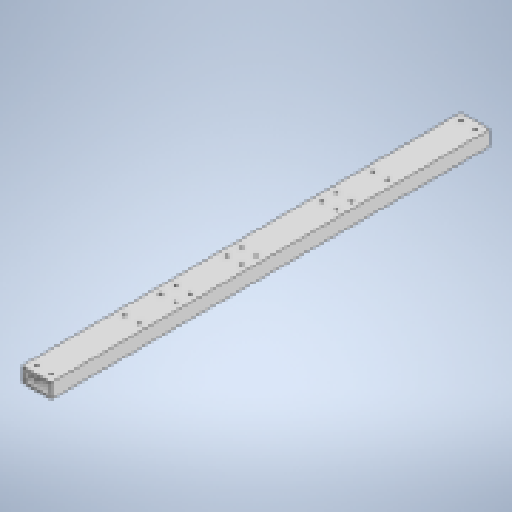
# Autodesk Inventor part: HorizontalSupportBar
Saved by Autodesk Inventor 2023 (Build 270158000, 158)
## iProperties
Created: 2022-07-13
Part Number: HorizontalSupportBar
Material: Generic
Document SubType Name: Modeling
Designer: Pratyush
Density: 1 g/cm^3
Appearance: Default
Author: Pratyush
Autodesk Inventor part; units mm, degrees
ref_plane "YZ Plane" through (0, 0, 0) normal (1, 0, 0) x (0, 1, 0)
ref_plane "XZ Plane" through (0, 0, 0) normal (0, 1, 0) x (-1, 0, 0)
ref_plane "XY Plane" through (0, 0, 0) normal (0, 0, 1) x (1, 0, 0)
sketch "Sketch1" plane through (0, 0, 0) normal (0, 0, 1) x (1, 0, 0)
  line L0 (-22.0343, 7.401) -> (28.7657, 7.401)
  line L1 (28.7657, 7.401) -> (28.7657, -17.999)
  line L2 (28.7657, -17.999) -> (-22.0343, -17.999)
  line L3 (-22.0343, -17.999) -> (-22.0343, 7.401)
  line L4 (-18.8593, 4.226) -> (25.5907, 4.226)
  line L5 (25.5907, 4.226) -> (25.5907, -14.824)
  line L6 (25.5907, -14.824) -> (-18.8593, -14.824)
  line L7 (-18.8593, -14.824) -> (-18.8593, 4.226)
  point P0 (0, 0)
  dimension "d0" = 50.8
  dimension "d1" = 25.4
  dimension "d2" = 3.175
  dimension "d3" = 3.175
  dimension "d4" = 3.175
  dimension "d5" = 3.175
  constraints: 16 end point, 4 parallel, 2 horizontal, 2 perpendicular
  measures "d0" distance of L0.start L0.end
  measures "d1" distance of L2.end L0.start
  measures "d2" distance between parallel lines of L0 L4
  measures "d3" distance between parallel lines of L2 L6
  measures "d4" distance between parallel lines of L1 L5
  measures "d5" distance between parallel lines of L3 L7
extrude "Extrusion1" add sketch "Sketch1" along normal mid plane 762
sketch "Sketch2" plane through (-22.0343, 7.401, 381) normal (0, 1, 0) x (1, 0, 0)
  line L0 (50.8, 0) -> (0, 0) projected
  line L1 (0, 762) -> (0, 0) projected
  point P0 (22.0343, 381)
  point P1 (12.7, 12.7)
  dimension "d8" = 12.7
  dimension "d9" = 12.7
  measures "d8" distance from line of L0 point (12.7, 12.7)
  measures "d9" distance from line of L1 point (12.7, 12.7)
hole "Hole1" at (-9.3343, 7.401, 368.3) direction (0, -1, 0) diameter 4.7625 depth 27.94
sketch "Sketch3" plane through (-22.0343, 7.401, 381) normal (0, 1, 0) x (1, 0, 0)
  line L0 (50.8, 0) -> (0, 0) projected
  line L1 (50.8, 762) -> (50.8, 0) projected
  point P0 (22.0343, 381)
  point P1 (38.1, 12.7)
  dimension "d17" = 12.7
  dimension "d18" = 12.7
  measures "d17" distance from line of L0 point (38.1, 12.7)
  measures "d18" distance from line of L1 point (38.1, 12.7)
hole "Hole2" at (16.0657, 7.401, 368.3) direction (0, -1, 0) diameter 4.7625 depth 27.94
sketch "Sketch4" plane through (-22.0343, 7.401, 381) normal (0, 1, 0) x (1, 0, 0)
  line L0 (0, 762) -> (0, 0) projected
  line L1 (50.8, 0) -> (0, 0) projected
  point P0 (22.0343, 381)
  point P1 (12.7, 165.1)
  dimension "d26" = 12.7
  dimension "d27" = 165.1
  measures "d26" distance from line of L0 point (12.7, 165.1)
  measures "d27" distance from line of L1 point (12.7, 165.1)
hole "Hole3" at (-9.3343, 7.401, 215.9) direction (0, -1, 0) diameter 4.7625 depth 27.94
sketch "Sketch5" plane through (-22.0343, 7.401, 381) normal (0, 1, 0) x (1, 0, 0)
  line L0 (50.8, 762) -> (50.8, 0) projected
  line L1 (50.8, 0) -> (0, 0) projected
  point P0 (22.0343, 381)
  point P1 (38.1, 165.1)
  dimension "d35" = 12.7
  dimension "d36" = 165.1
  measures "d35" distance from line of L0 point (38.1, 165.1)
  measures "d36" distance from line of L1 point (38.1, 165.1)
hole "Hole4" at (16.0657, 7.401, 215.9) direction (0, -1, 0) diameter 4.7625 depth 27.94
sketch "Sketch6" plane through (-22.0343, 7.401, 381) normal (0, 1, 0) x (1, 0, 0)
  line L0 (0, 762) -> (50.8, 762) projected
  line L1 (0, 762) -> (0, 0) projected
  point P0 (22.0343, 381)
  point P1 (12.7, 749.3)
  dimension "d44" = 12.7
  dimension "d45" = 12.7
  measures "d44" distance from line of L0 point (12.7, 749.3)
  measures "d45" distance from line of L1 point (12.7, 749.3)
hole "Hole5" at (-9.3343, 7.401, -368.3) direction (0, -1, 0) diameter 4.7625 depth 27.94
sketch "Sketch7" plane through (-22.0343, 7.401, 381) normal (0, 1, 0) x (1, 0, 0)
  line L0 (0, 762) -> (50.8, 762) projected
  line L1 (50.8, 762) -> (50.8, 0) projected
  point P0 (22.0343, 381)
  point P1 (38.1, 749.3)
  dimension "d53" = 12.7
  dimension "d54" = 12.7
  measures "d53" distance from line of L0 point (38.1, 749.3)
  measures "d54" distance from line of L1 point (38.1, 749.3)
hole "Hole6" at (16.0657, 7.401, -368.3) direction (0, -1, 0) diameter 4.7625 depth 27.94
sketch "Sketch8" plane through (-22.0343, 7.401, 381) normal (0, 1, 0) x (1, 0, 0)
  line L0 (0, 762) -> (50.8, 762) projected
  line L1 (0, 762) -> (0, 0) projected
  point P0 (22.0343, 381)
  point P1 (12.7, 596.9)
  dimension "d62" = 165.1
  dimension "d63" = 12.7
  measures "d62" distance from line of L0 point (12.7, 596.9)
  measures "d63" distance from line of L1 point (12.7, 596.9)
hole "Hole7" at (-9.3343, 7.401, -215.9) direction (0, -1, 0) diameter 4.7625 depth 27.94
sketch "Sketch9" plane through (-22.0343, 7.401, 381) normal (0, 1, 0) x (1, 0, 0)
  line L0 (0, 762) -> (50.8, 762) projected
  line L1 (50.8, 762) -> (50.8, 0) projected
  point P0 (22.0343, 381)
  point P1 (38.1, 596.9)
  dimension "d71" = 165.1
  dimension "d72" = 12.7
  measures "d71" distance from line of L0 point (38.1, 596.9)
  measures "d72" distance from line of L1 point (38.1, 596.9)
hole "Hole8" at (16.0657, 7.401, -215.9) direction (0, -1, 0) diameter 4.7625 depth 27.94
sketch "Sketch14" plane through (-22.0343, 7.401, 381) normal (0, 1, 0) x (1, 0, 0)
  line L0 (0, 762) -> (0, 0) projected
  line L1 (50.8, 0) -> (0, 0) projected
  point P0 (22.0343, 381)
  point P1 (12.7, 254)
  dimension "d116" = 12.7
  dimension "d117" = 254
  measures "d116" distance from line of L0 point (12.7, 254)
  measures "d117" distance from line of L1 point (12.7, 254)
hole "Hole13" at (-9.3343, 7.401, 127) direction (0, -1, 0) diameter 4.7625 depth 104.14
sketch "Sketch15" plane through (-22.0343, 7.401, 381) normal (0, 1, 0) x (1, 0, 0)
  line L0 (0, 762) -> (0, 0) projected
  line L1 (50.8, 0) -> (0, 0) projected
  point P0 (22.0343, 381)
  point P1 (38.1, 254)
  dimension "d125" = 38.1
  dimension "d126" = 254
  measures "d125" distance from line of L0 point (38.1, 254)
  measures "d126" distance from line of L1 point (38.1, 254)
hole "Hole14" at (16.0657, 7.401, 127) direction (0, -1, 0) diameter 4.7625 depth 104.14
sketch "Sketch16" plane through (-22.0343, 7.401, 381) normal (0, 1, 0) x (1, 0, 0)
  line L0 (0, 762) -> (0, 0) projected
  line L1 (50.8, 0) -> (0, 0) projected
  point P0 (22.0343, 381)
  point P1 (12.7, 228.6)
  dimension "d134" = 12.7
  dimension "d135" = 228.6
  measures "d134" distance from line of L0 point (12.7, 228.6)
  measures "d135" distance from line of L1 point (12.7, 228.6)
hole "Hole15" at (-9.3343, 7.401, 152.4) direction (0, -1, 0) diameter 4.7625 depth 104.14
sketch "Sketch17" plane through (-22.0343, 7.401, 381) normal (0, 1, 0) x (1, 0, 0)
  line L0 (50.8, 0) -> (0, 0) projected
  line L1 (50.8, 762) -> (50.8, 0) projected
  point P0 (22.0343, 381)
  point P1 (38.1, 228.6)
  dimension "d143" = 228.6
  dimension "d144" = 12.7
  measures "d143" distance from line of L0 point (38.1, 228.6)
  measures "d144" distance from line of L1 point (38.1, 228.6)
hole "Hole16" at (16.0657, 7.401, 152.4) direction (0, -1, 0) diameter 4.7625 depth 104.14
sketch "Sketch18" plane through (-22.0343, -17.999, 381) normal (0, -1, 0) x (1, 0, 0)
  line L0 (50.8, -762) -> (50.8, 0) projected
  line L1 (0, 0) -> (50.8, 0) projected
  point P0 (22.0343, -381)
  point P1 (38.1, -342.9)
  dimension "d152" = 12.7
  dimension "d153" = 342.9
  measures "d152" distance from line of L0 point (38.1, -342.9)
  measures "d153" distance from line of L1 point (38.1, -342.9)
hole "Hole17" at (16.0657, -17.999, 38.1) direction (0, 1, 0) diameter 4.7625 depth 104.14
sketch "Sketch19" plane through (-22.0343, -17.999, 381) normal (0, -1, 0) x (1, 0, 0)
  line L0 (0, 0) -> (0, -762) projected
  line L1 (0, 0) -> (50.8, 0) projected
  point P0 (22.0343, -381)
  point P1 (12.7, -342.9)
  dimension "d161" = 12.7
  dimension "d162" = 342.9
  measures "d161" distance from line of L0 point (12.7, -342.9)
  measures "d162" distance from line of L1 point (12.7, -342.9)
hole "Hole18" at (-9.3343, -17.999, 38.1) direction (0, 1, 0) diameter 4.7625 depth 104.14
sketch "Sketch20" plane through (-22.0343, -17.999, 381) normal (0, -1, 0) x (1, 0, 0)
  line L0 (50.8, -762) -> (50.8, 0) projected
  line L1 (50.8, -762) -> (0, -762) projected
  point P0 (22.0343, -381)
  point P1 (38.1, -368.3)
  dimension "d170" = 12.7
  dimension "d171" = 393.7
  measures "d170" distance from line of L0 point (38.1, -368.3)
  measures "d171" distance from line of L1 point (38.1, -368.3)
hole "Hole19" at (16.0657, -17.999, 12.7) direction (0, 1, 0) diameter 4.7625 depth 104.14
sketch "Sketch21" plane through (-22.0343, -17.999, 381) normal (0, -1, 0) x (1, 0, 0)
  line L0 (50.8, -762) -> (50.8, 0) projected
  line L1 (50.8, -762) -> (0, -762) projected
  point P0 (22.0343, -381)
  point P1 (12.7, -368.3)
  dimension "d179" = 38.1
  dimension "d180" = 393.7
  measures "d179" distance from line of L0 point (12.7, -368.3)
  measures "d180" distance from line of L1 point (12.7, -368.3)
hole "Hole20" at (-9.3343, -17.999, 12.7) direction (0, 1, 0) diameter 4.7625 depth 104.14
equation "\"d4\" = d3"
equation "\"d5\" = d3"
body "Solid1"
